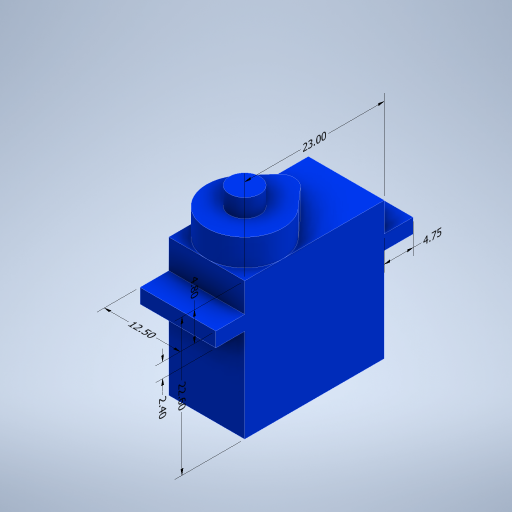
# Autodesk Inventor part: sg90_Tower_Pro
Saved by Autodesk Inventor 2024.1 (Build 281209000, 209)
## iProperties
Created: 2025-01-10
Part Number: sg90_Tower_Pro
Material: 一般
Document SubType Name: Modeling
Designer: hibik
Density: 1 g/cm^3
Appearance: 既定
Author: hibik
Autodesk Inventor part; units mm, degrees
ref_plane "YZ Plane" through (0, 0, 0) normal (1, 0, 0) x (0, 1, 0)
ref_plane "XZ Plane" through (0, 0, 0) normal (0, 1, 0) x (-1, 0, 0)
sketch "スケッチ1" plane through (0, 0, 0) normal (0, 1, 0) x (-1, 0, 0)
  line L0 (6.25, -16.75) -> (-6.25, -16.75)
  line L1 (-6.25, -16.75) -> (-6.25, 6.25)
  line L2 (-6.25, 6.25) -> (6.25, 6.25)
  line L3 (6.25, 6.25) -> (6.25, -16.75)
  line L4 (6.25, -16.75) -> (-6.25, 6.25) construction
  line L5 (-6.25, -16.75) -> (6.25, 6.25) construction
  point P0 (0, 0)
  point P1 (0, -5.25)
  dimension "d0" = 12.5
  dimension "d1" = 23
  dimension "d2" = 6.25
  constraints: 12 end point, 2 midpoint, 2 parallel, 1 horizontal, 1 perpendicular, 1 vertical alignment
  measures "d0" distance of L1.end L2.end
  measures "d1" distance of L0.end L1.end
  measures "d2" distance from line of point (0, 0) L2
extrude "押し出し1" add sketch "スケッチ1" along normal blind 22.6
sketch "スケッチ2" plane through (0, 22.6, 0) normal (0, 1, 0) x (1, 0, 0)
  circle A0 centre (0, 0) radius 6.25
  line L0 (-6.25, -6.25) -> (6.25, -6.25) projected
  line L1 (6.25, -6.25) -> (6.25, 16.75) projected
  line L2 (-6.25, 16.75) -> (-6.25, -6.25) projected
  circle A1 centre (0, 5.65) radius 2.5
  line L3 (-1.87, 7.3093) -> (-4.6749, 4.1482)
  line L4 (1.87, 7.3093) -> (4.6749, 4.1482)
  point P0 (0, 0)
  point P1 (-2.4988, 5.7288)
  point P2 (2.4988, 5.7288)
  dimension "d14" = 5
  dimension "d33" = 11.9
  constraints: 7 tangent, 4 end point, 4 point on circle, 2 centre point, 1 vertical alignment
  measures "d14" diameter of A1
  measures "d33" distance from line of L0 A1.centre
extrude "押し出し2" add sketch "スケッチ2" along normal blind 4.4 contours A0 A1 | A0 A1 L4 | A1 A0 | A0 A1 | A0 L3 A1
ref_plane "作業平面1" through (0, 15.4, 0) normal (0, -1, 0) x (1, 0, 0)
sketch "スケッチ3" plane through (0, 15.4, 0) normal (0, -1, 0) x (1, 0, 0)
  line L0 (-6.25, 11) -> (6.25, 11)
  line L1 (6.25, 11) -> (6.25, -21.5)
  line L2 (6.25, -21.5) -> (-6.25, -21.5)
  line L3 (-6.25, -21.5) -> (-6.25, 11)
  line L4 (-6.25, 11) -> (6.25, -21.5) construction
  line L5 (6.25, 11) -> (-6.25, -21.5) construction
  line L6 (-6.25, 0) -> (-6.25, 6.25) projected
  line L7 (6.25, 0) -> (6.25, -16.75) projected
  line L8 (-6.25, -16.75) -> (-6.25, 6.25) projected
  point P0 (0, 0)
  point P1 (0, -5.25)
  point P2 (-6.25, -5.25)
  dimension "d8" = 32.5
  constraints: 12 end point, 4 midpoint, 2 collinear, 2 parallel, 1 horizontal, 1 perpendicular
  measures "d8" distance of L0.end L1.end
extrude "押し出し3" add sketch "スケッチ3" against normal blind 2.4
sketch "スケッチ4" plane through (0, 27, 0) normal (0, 1, 0) x (1, 0, 0)
  circle A0 centre (0, 0) radius 2.5
  point P0 (0, 0)
  dimension "d11" = 5
  constraints: 1 centre point, 1 coincident
  measures "d11" diameter of A0
extrude "押し出し4" add sketch "スケッチ4" along normal blind 3
